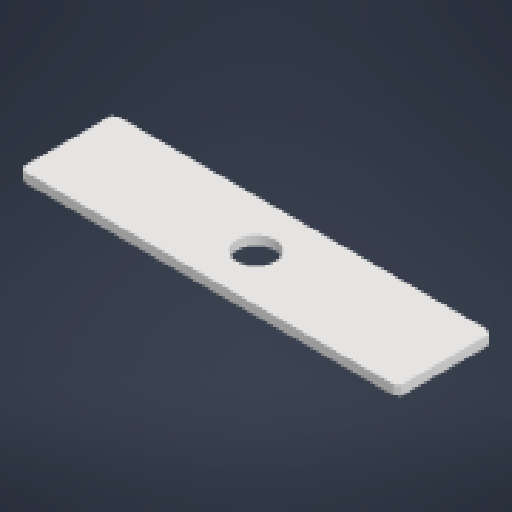
# Autodesk Inventor part: rig_connector
Saved by Autodesk Inventor 2027.1 (Build 311270010, 270A)
## iProperties
Created: 2026-09-04
Part Number: rig_connector
Material: Generic
Document SubType Name: Modeling
Designer: ajrcr
Density: 1 g/cm^3
Appearance: Default
Author: ajrcr
Autodesk Inventor part; units mm, degrees
ref_plane "YZ Plane" through (0, 0, 0) normal (1, 0, 0) x (0, 1, 0)
ref_plane "XZ Plane" through (0, 0, 0) normal (0, 1, 0) x (-1, 0, 0)
ref_plane "XY Plane" through (0, 0, 0) normal (0, 0, 1) x (1, 0, 0)
sketch "Sketch1" plane through (0, 0, 0) normal (0, 1, 0) x (-1, 0, 0)
  line L0 (-58.5, -15) -> (58.5, -15)
  line L1 (60, -14) -> (60, 14)
  line L2 (58.5, 15) -> (-58.5, 15)
  line L3 (-60, 14) -> (-60, -14)
  circle A0 centre (0, 0) radius 6
  line L4 (-58.5, -15) -> (-60, -14)
  line L5 (-60, 14) -> (-58.5, 15)
  line L6 (60, 14) -> (58.5, 15)
  line L7 (60, -14) -> (58.5, -15)
  point P0 (-60, -15)
  point P1 (60, 15)
  point P2 (60, -15)
  point P3 (-60, 15)
  point P4 (60, 0)
  dimension "d0" = 120
  dimension "d1" = 30
  dimension "d2" = 60
  dimension "d3" = 15
  dimension "d6" = 12
  dimension "d7" = 1.5
  dimension "d8" = 1
  dimension "d9" = 1
  dimension "d10" = 1.5
  dimension "d11" = 1
  dimension "d12" = 1.5
  dimension "d13" = 1
  dimension "d14" = 1.5
  constraints: 16 end point, 8 point on line, 2 parallel, 1 centre point, 1 coincident, 1 horizontal, 1 midpoint, 1 perpendicular
  measures "d0" distance of point (-60, 15) point (60, 15)
  measures "d1" distance of point (60, 15) point (60, -15)
  measures "d2" distance of point (0, 0) point (60, 0)
  measures "d3" distance from line of L0 point (0, 0)
  measures "d6" diameter of A0
  measures "d7" distance of L0.start point (-60, -15)
  measures "d8" distance of L3.end point (-60, -15)
  measures "d9" distance of L3.start point (-60, 15)
  measures "d10" distance of L2.end point (-60, 15)
  measures "d11" distance of L1.end point (60, 15)
  measures "d12" distance of L2.start point (60, 15)
  measures "d13" distance of L1.start point (60, -15)
  measures "d14" distance of L0.end point (60, -15)
extrude "Extrusion1" add sketch "Sketch1" along normal blind 3
equation "\"d9\" = d8"
equation "\"d10\" = d7"
equation "\"d11\" = d8"
equation "\"d12\" = d7"
equation "\"d13\" = d8"
equation "\"d14\" = d7"
body "Solid1"
